Autodesk Fusion 360 part; units mm, degrees
note: some values were not read from the file. Chosen so that the rebuilt part matches the saved one: which bodies a step acts on. Set by a fixed rule: which sketch regions a step uses.
(part 5 of 6)
  point P38 (-7.0016, 32.4227)
  point P39 (-7.9355, 32.3003)
  point P40 (-6.6625, 36.7231)
  point P41 (-7.4801, 35.8372)
  point P42 (-8.2403, 35.0791)
  point P43 (-8.9343, 34.4424)
  point P44 (-7.8535, 39.011)
  point P45 (-9.0481, 38.8495)
  point P46 (-10.1052, 38.6615)
  point P47 (-11.0249, 38.4582)
  point P48 (-10.1422, 42.9752)
  point P49 (-10.8794, 42.0214)
  point P50 (-11.5708, 41.1999)
  point P51 (-12.2066, 40.5051)
  point P52 (-11.5281, 45.1505)
  point P53 (-12.7041, 44.8855)
  point P54 (-13.7407, 44.6061)
  point P55 (-14.6392, 44.3235)
  point P56 (-14.1536, 48.9001)
  point P57 (-14.8049, 47.8857)
  point P58 (-15.422, 47.0071)
  point P59 (-15.9948, 46.2596)
  point P60 (-15.7238, 50.9464)
  point P61 (-16.8722, 50.5799)
  point P62 (-17.8806, 50.2113)
  point P63 (-18.7509, 49.8514)
  point P64 (-18.6661, 54.453)
  point P65 (-19.2265, 53.3857)
  point P66 (-19.7646, 52.4566)
  point P67 (-20.2702, 51.6619)
  point P68 (-20.4086, 56.3546)
  point P69 (-21.5207, 55.8894)
  point P70 (-22.4931, 55.4343)
  point P71 (-23.3289, 54.9999)
  point P72 (-23.6454, 59.5914)
  point P73 (-24.1106, 58.4793)
  point P74 (-24.5657, 57.5069)
  point P75 (-25.0001, 56.6711)
  point P76 (-25.547, 61.3339)
  point P77 (-26.6143, 60.7735)
  point P78 (-27.5434, 60.2354)
  point P79 (-28.3381, 59.7298)
  point P80 (-29.0536, 64.2762)
  point P81 (-29.4201, 63.1278)
  point P82 (-29.7887, 62.1194)
  point P83 (-30.1486, 61.2491)
  point P84 (-31.0999, 65.8464)
  point P85 (-32.1143, 65.1951)
  point P86 (-32.9929, 64.578)
  point P87 (-33.7404, 64.0052)
  point P88 (-34.8495, 68.4719)
  point P89 (-35.1145, 67.2959)
  point P90 (-35.3939, 66.2593)
  point P91 (-35.6765, 65.3608)
  point P92 (-37.0248, 69.8578)
  point P93 (-37.9786, 69.1206)
  point P94 (-38.8001, 68.4292)
  point P95 (-39.4949, 67.7934)
  point P96 (-40.989, 72.1465)
  point P97 (-41.1505, 70.9519)
  point P98 (-41.3385, 69.8948)
  point P99 (-41.5418, 68.9751)
  point P100 (-43.2769, 73.3375)
  point P101 (-44.1628, 72.5199)
  point P102 (-44.9209, 71.7597)
  point P103 (-45.5576, 71.0657)
  point P104 (-47.4254, 75.272)
  point P105 (-47.4822, 74.0678)
  point P106 (-47.5773, 72.9984)
  point P107 (-47.6997, 72.0645)
  point P108 (-49.8084, 76.259)
  point P109 (-50.6197, 75.3674)
  point P110 (-51.3086, 74.5439)
  point P111 (-51.8825, 73.7971)
  point P112 (-54.1098, 77.8246)
  point P113 (-54.0614, 76.6201)
  point P114 (-54.063, 75.5464)
  point P115 (-54.1034, 74.6055)
  point P116 (-56.5697, 78.6002)
  point P117 (-57.3002, 77.6413)
  point P118 (-57.9147, 76.7609)
  point P119 (-58.4213, 75.9669)
  point P120 (-60.9911, 79.7849)
  point P121 (-60.838, 78.5892)
  point P122 (-60.746, 77.5195)
  point P123 (-60.7043, 76.5786)
  point P124 (-63.5093, 80.3432)
  point P125 (-64.1534, 79.3242)
  point P126 (-64.6889, 78.3937)
  point P127 (-65.1244, 77.5585)
  point P128 (-68.0172, 81.1381)
  point P129 (-67.7604, 79.9603)
  point P130 (-67.5755, 78.9026)
  point P131 (-67.452, 77.9689)
  point P132 (-70.5744, 81.4747)
  point P133 (-71.1273, 80.4035)
  point P134 (-71.5796, 79.4298)
  point P135 (-71.9406, 78.5599)
  point P136 (-75.1344, 81.8737)
  point P137 (-74.776, 80.7227)
  point P138 (-74.4996, 79.6853)
  point P139 (-74.2952, 78.7659)
  point P140 (-77.7113, 81.9862)
  point P141 (-78.1687, 80.8709)
  point P142 (-78.5345, 79.8614)
  point P143 (-78.8182, 78.9633)
  point P144 (-82.2887, 81.9862)
  point P145 (-81.8313, 80.8709)
  point P146 (-81.4655, 79.8614)
  point P147 (-81.1818, 78.9633)
  point P148 (-84.8656, 81.8737)
  point P149 (-85.224, 80.7227)
  point P150 (-85.5004, 79.6853)
  point P151 (-85.7048, 78.7659)
  point P152 (-89.4256, 81.4747)
  point P153 (-88.8727, 80.4035)
  point P154 (-88.4204, 79.4298)
  point P155 (-88.0594, 78.5599)
  point P156 (-91.9828, 81.1381)
  point P157 (-92.2396, 79.9603)
  point P158 (-92.4245, 78.9026)
  point P159 (-92.548, 77.9689)
  point P160 (-96.4907, 80.3432)
  point P161 (-95.8466, 79.3242)
  point P162 (-95.3111, 78.3937)
  point P163 (-94.8756, 77.5585)
  point P164 (-99.0089, 79.7849)
  point P165 (-99.162, 78.5892)
  point P166 (-99.254, 77.5195)
  point P167 (-99.2957, 76.5786)
  point P168 (-103.4303, 78.6002)
  point P169 (-102.6998, 77.6413)
  point P170 (-102.0853, 76.7609)
  point P171 (-101.5787, 75.9669)
  point P172 (-105.8902, 77.8246)
  point P173 (-105.9386, 76.6201)
  point P174 (-105.937, 75.5464)
  point P175 (-105.8966, 74.6055)
  point P176 (-110.1916, 76.259)
  point P177 (-109.3803, 75.3674)
  point P178 (-108.6914, 74.5439)
  point P179 (-108.1175, 73.7971)
  point P180 (-112.5746, 75.272)
  point P181 (-112.5178, 74.0678)
  point P182 (-112.4227, 72.9984)
  point P183 (-112.3003, 72.0645)
  point P184 (-116.7231, 73.3375)
  point P185 (-115.8372, 72.5199)
  point P186 (-115.0791, 71.7597)
  point P187 (-114.4424, 71.0657)
  point P188 (-119.011, 72.1465)
  point P189 (-118.8495, 70.9519)
  point P190 (-118.6615, 69.8948)
  point P191 (-118.4582, 68.9751)
  point P192 (-122.9752, 69.8578)
  point P193 (-122.0214, 69.1206)
  point P194 (-121.1999, 68.4292)
  point P195 (-120.5051, 67.7934)
  point P196 (-125.1505, 68.4719)
  point P197 (-124.8855, 67.2959)
  point P198 (-124.6061, 66.2593)
  point P199 (-124.3235, 65.3608)
  point P200 (-128.9001, 65.8464)
  point P201 (-127.8857, 65.1951)
  point P202 (-127.0071, 64.578)
  point P203 (-126.2596, 64.0052)
  point P204 (-130.9464, 64.2762)
  point P205 (-130.5799, 63.1278)
  point P206 (-130.2113, 62.1194)
  point P207 (-129.8514, 61.2491)
  point P208 (-134.453, 61.3339)
  point P209 (-133.3857, 60.7735)
  point P210 (-132.4566, 60.2354)
  point P211 (-131.6619, 59.7298)
  point P212 (-136.3546, 59.5914)
  point P213 (-135.8894, 58.4793)
  point P214 (-135.4343, 57.5069)
  point P215 (-134.9999, 56.6711)
  point P216 (-139.5914, 56.3546)
  point P217 (-138.4793, 55.8894)
  point P218 (-137.5069, 55.4343)
  point P219 (-136.6711, 54.9999)
  point P220 (-141.3339, 54.453)
  point P221 (-140.7735, 53.3857)
  point P222 (-140.2354, 52.4566)
  point P223 (-139.7298, 51.6619)
  point P224 (-144.2762, 50.9464)
  point P225 (-143.1278, 50.5799)
  point P226 (-142.1194, 50.2113)
  point P227 (-141.2491, 49.8514)
  point P228 (-145.8464, 48.9001)
  point P229 (-145.1951, 47.8857)
  point P230 (-144.578, 47.0071)
  point P231 (-144.0052, 46.2596)
  point P232 (-148.4719, 45.1505)
  point P233 (-147.2959, 44.8855)
  point P234 (-146.2593, 44.6061)
  point P235 (-145.3608, 44.3235)
  point P236 (-149.8578, 42.9752)
  point P237 (-149.1206, 42.0214)
  point P238 (-148.4292, 41.1999)
  point P239 (-147.7934, 40.5051)
  point P240 (-152.1465, 39.011)
  point P241 (-150.9519, 38.8495)
  point P242 (-149.8948, 38.6615)
  point P243 (-148.9751, 38.4582)
  point P244 (-153.3375, 36.7231)
  point P245 (-152.5199, 35.8372)
  point P246 (-151.7597, 35.0791)
  point P247 (-151.0657, 34.4424)
  point P248 (-155.272, 32.5746)
  point P249 (-154.0678, 32.5178)
  point P250 (-152.9984, 32.4227)
  point P251 (-152.0645, 32.3003)
  point P252 (-156.259, 30.1916)
  point P253 (-155.3674, 29.3803)
  point P254 (-154.5439, 28.6914)
  point P255 (-153.7971, 28.1175)
  point P256 (-157.8246, 25.8902)
  point P257 (-156.6201, 25.9386)
  point P258 (-155.5464, 25.937)
  point P259 (-154.6055, 25.8966)
  point P260 (-158.6002, 23.4303)
  point P261 (-157.6413, 22.6998)
  point P262 (-156.7609, 22.0853)
  point P263 (-155.9669, 21.5787)
  point P264 (-159.7849, 19.0089)
  point P265 (-158.5892, 19.162)
  point P266 (-157.5195, 19.254)
  point P267 (-156.5786, 19.2957)
  point P268 (-160.3432, 16.4907)
  point P269 (-159.3242, 15.8466)
  point P270 (-158.3937, 15.3111)
  point P271 (-157.5585, 14.8756)
  point P272 (-161.1381, 11.9828)
  point P273 (-159.9603, 12.2396)
  point P274 (-158.9026, 12.4245)
  point P275 (-157.9689, 12.548)
  point P276 (-161.4747, 9.4256)
  point P277 (-160.4035, 8.8727)
  point P278 (-159.4298, 8.4204)
  point P279 (-158.5599, 8.0594)
  point P280 (-161.8737, 4.8656)
  point P281 (-160.7227, 5.224)
  point P282 (-159.6853, 5.5004)
  point P283 (-158.7659, 5.7048)
  point P284 (-161.9862, 2.2887)
  point P285 (-160.8709, 1.8313)
  point P286 (-159.8614, 1.4655)
  point P287 (-158.9633, 1.1818)
  point P288 (-161.9862, -2.2887)
  point P289 (-160.8709, -1.8313)
  point P290 (-159.8614, -1.4655)
  point P291 (-158.9633, -1.1818)
  point P292 (-161.8737, -4.8656)
  point P293 (-160.7227, -5.224)
  point P294 (-159.6853, -5.5004)
  point P295 (-158.7659, -5.7048)
  point P296 (-161.4747, -9.4256)
  point P297 (-160.4035, -8.8727)
  point P298 (-159.4298, -8.4204)
  point P299 (-158.5599, -8.0594)
  point P300 (-161.1381, -11.9828)
  point P301 (-159.9603, -12.2396)
  point P302 (-158.9026, -12.4245)
  point P303 (-157.9689, -12.548)
  point P304 (-160.3432, -16.4907)
  point P305 (-159.3242, -15.8466)
  point P306 (-158.3937, -15.3111)
  point P307 (-157.5585, -14.8756)
  point P308 (-159.7849, -19.0089)
  point P309 (-158.5892, -19.162)
  point P310 (-157.5195, -19.254)
  point P311 (-156.5786, -19.2957)
  point P312 (-158.6002, -23.4303)
  point P313 (-157.6413, -22.6998)
  point P314 (-156.7609, -22.0853)
  point P315 (-155.9669, -21.5787)
  point P316 (-157.8246, -25.8902)
  point P317 (-156.6201, -25.9386)
  point P318 (-155.5464, -25.937)
  point P319 (-154.6055, -25.8966)
  point P320 (-156.259, -30.1916)
  point P321 (-155.3674, -29.3803)
  point P322 (-154.5439, -28.6914)
  point P323 (-153.7971, -28.1175)
  point P324 (-155.272, -32.5746)
  point P325 (-154.0678, -32.5178)
  point P326 (-152.9984, -32.4227)
  point P327 (-152.0645, -32.3003)
  point P328 (-153.3375, -36.7231)
  point P329 (-152.5199, -35.8372)
  point P330 (-151.7597, -35.0791)
  point P331 (-151.0657, -34.4424)
  point P332 (-152.1465, -39.011)
  point P333 (-150.9519, -38.8495)
  point P334 (-149.8948, -38.6615)
  point P335 (-148.9751, -38.4582)
  point P336 (-149.8578, -42.9752)
  point P337 (-149.1206, -42.0214)
  point P338 (-148.4292, -41.1999)
  point P339 (-147.7934, -40.5051)
  point P340 (-148.4719, -45.1505)
  point P341 (-147.2959, -44.8855)
  point P342 (-146.2593, -44.6061)
  point P343 (-145.3608, -44.3235)
  point P344 (-145.8464, -48.9001)
  point P345 (-145.1951, -47.8857)
  point P346 (-144.578, -47.0071)
  point P347 (-144.0052, -46.2596)
  point P348 (-144.2762, -50.9464)
  point P349 (-143.1278, -50.5799)
  point P350 (-142.1194, -50.2113)
  point P351 (-141.2491, -49.8514)
  point P352 (-141.3339, -54.453)
  point P353 (-140.7735, -53.3857)
  point P354 (-140.2354, -52.4566)
  point P355 (-139.7298, -51.6619)
  point P356 (-139.5914, -56.3546)
  point P357 (-138.4793, -55.8894)
  point P358 (-137.5069, -55.4343)
  point P359 (-136.6711, -54.9999)
  point P360 (-136.3546, -59.5914)
  point P361 (-135.8894, -58.4793)
  point P362 (-135.4343, -57.5069)
  point P363 (-134.9999, -56.6711)
  point P364 (-134.453, -61.3339)
  point P365 (-133.3857, -60.7735)
  point P366 (-132.4566, -60.2354)
  point P367 (-131.6619, -59.7298)
  point P368 (-130.9464, -64.2762)
  point P369 (-130.5799, -63.1278)
  point P370 (-130.2113, -62.1194)
  point P371 (-129.8514, -61.2491)
  point P372 (-128.9001, -65.8464)
  point P373 (-127.8857, -65.1951)
  point P374 (-127.0071, -64.578)
  point P375 (-126.2596, -64.0052)
  point P376 (-125.1505, -68.4719)
  point P377 (-124.8855, -67.2959)
  point P378 (-124.6061, -66.2593)
  point P379 (-124.3235, -65.3608)
  point P380 (-122.9752, -69.8578)
  point P381 (-122.0214, -69.1206)
  point P382 (-121.1999, -68.4292)
  point P383 (-120.5051, -67.7934)
  point P384 (-119.011, -72.1465)
  point P385 (-118.8495, -70.9519)
  point P386 (-118.6615, -69.8948)
  point P387 (-118.4582, -68.9751)
  point P388 (-116.7231, -73.3375)
  point P389 (-115.8372, -72.5199)
  point P390 (-115.0791, -71.7597)
  point P391 (-114.4424, -71.0657)
  point P392 (-112.5746, -75.272)
  point P393 (-112.5178, -74.0678)
  point P394 (-112.4227, -72.9984)
  point P395 (-112.3003, -72.0645)
  point P396 (-110.1916, -76.259)
  point P397 (-109.3803, -75.3674)
  point P398 (-108.6914, -74.5439)
  point P399 (-108.1175, -73.7971)
  point P400 (-105.8902, -77.8246)
  point P401 (-105.9386, -76.6201)
  point P402 (-105.937, -75.5464)
  point P403 (-105.8966, -74.6055)
  point P404 (-103.4303, -78.6002)
  point P405 (-102.6998, -77.6413)
  point P406 (-102.0853, -76.7609)
  point P407 (-101.5787, -75.9669)
  point P408 (-99.0089, -79.7849)
  point P409 (-99.162, -78.5892)
  point P410 (-99.254, -77.5195)
  point P411 (-99.2957, -76.5786)
  point P412 (-96.4907, -80.3432)
  point P413 (-95.8466, -79.3242)
  point P414 (-95.3111, -78.3937)
  point P415 (-94.8756, -77.5585)
  point P416 (-91.9828, -81.1381)
  point P417 (-92.2396, -79.9603)
  point P418 (-92.4245, -78.9026)
  point P419 (-92.548, -77.9689)
  point P420 (-89.4256, -81.4747)
  point P421 (-88.8727, -80.4035)
  point P422 (-88.4204, -79.4298)
  point P423 (-88.0594, -78.5599)
  point P424 (-84.8656, -81.8737)
  point P425 (-85.224, -80.7227)
  point P426 (-85.5004, -79.6853)
  point P427 (-85.7048, -78.7659)
  point P428 (-82.2887, -81.9862)
  point P429 (-81.8313, -80.8709)
  point P430 (-81.4655, -79.8614)
  point P431 (-81.1818, -78.9633)
  point P432 (-77.7113, -81.9862)
  point P433 (-78.1687, -80.8709)
  point P434 (-78.5345, -79.8614)
  point P435 (-78.8182, -78.9633)
  point P436 (-75.1344, -81.8737)
  point P437 (-74.776, -80.7227)
  point P438 (-74.4996, -79.6853)
  point P439 (-74.2952, -78.7659)
  point P440 (-70.5744, -81.4747)
  point P441 (-71.1273, -80.4035)
  point P442 (-71.5796, -79.4298)
  point P443 (-71.9406, -78.5599)
  point P444 (-68.0172, -81.1381)
  point P445 (-67.7604, -79.9603)
  point P446 (-67.5755, -78.9026)
  point P447 (-67.452, -77.9689)
  point P448 (-63.5093, -80.3432)
  point P449 (-64.1534, -79.3242)
  point P450 (-64.6889, -78.3937)
  point P451 (-65.1244, -77.5585)
  point P452 (-60.9911, -79.7849)
  point P453 (-60.838, -78.5892)
  point P454 (-60.746, -77.5195)
  point P455 (-60.7043, -76.5786)
  point P456 (-56.5697, -78.6002)
  point P457 (-57.3002, -77.6413)
  point P458 (-57.9147, -76.7609)
  point P459 (-58.4213, -75.9669)
  point P460 (-54.1098, -77.8246)
  point P461 (-54.0614, -76.6201)
  point P462 (-54.063, -75.5464)
  point P463 (-54.1034, -74.6055)
  point P464 (-49.8084, -76.259)
  point P465 (-50.6197, -75.3674)
  point P466 (-51.3086, -74.5439)
  point P467 (-51.8825, -73.7971)
  point P468 (-47.4254, -75.272)
  point P469 (-47.4822, -74.0678)
  point P470 (-47.5773, -72.9984)
  point P471 (-47.6997, -72.0645)
  point P472 (-43.2769, -73.3375)
  point P473 (-44.1628, -72.5199)
  point P474 (-44.9209, -71.7597)
  point P475 (-45.5576, -71.0657)
  point P476 (-40.989, -72.1465)
  point P477 (-41.1505, -70.9519)
  point P478 (-41.3385, -69.8948)
  point P479 (-41.5418, -68.9751)
  point P480 (-37.0248, -69.8578)
  point P481 (-37.9786, -69.1206)
  point P482 (-38.8001, -68.4292)
  point P483 (-39.4949, -67.7934)
  point P484 (-34.8495, -68.4719)
  point P485 (-35.1145, -67.2959)
  point P486 (-35.3939, -66.2593)
  point P487 (-35.6765, -65.3608)
  point P488 (-31.0999, -65.8464)
  point P489 (-32.1143, -65.1951)
  point P490 (-32.9929, -64.578)
  point P491 (-33.7404, -64.0052)
  point P492 (-29.0536, -64.2762)
  point P493 (-29.4201, -63.1278)
  point P494 (-29.7887, -62.1194)
  point P495 (-30.1486, -61.2491)
  point P496 (-25.547, -61.3339)
  point P497 (-26.6143, -60.7735)
  point P498 (-27.5434, -60.2354)
  point P499 (-28.3381, -59.7298)
  point P500 (-23.6454, -59.5914)
  point P501 (-24.1106, -58.4793)
  point P502 (-24.5657, -57.5069)
  point P503 (-25.0001, -56.6711)
  point P504 (-20.4086, -56.3546)
  point P505 (-21.5207, -55.8894)
  point P506 (-22.4931, -55.4343)
  point P507 (-23.3289, -54.9999)
  point P508 (-18.6661, -54.453)
  point P509 (-19.2265, -53.3857)
  point P510 (-19.7646, -52.4566)
  point P511 (-20.2702, -51.6619)
  point P512 (-15.7238, -50.9464)
  point P513 (-16.8722, -50.5799)
  point P514 (-17.8806, -50.2113)
  point P515 (-18.7509, -49.8514)
  point P516 (-14.1536, -48.9001)
  point P517 (-14.8049, -47.8857)
  point P518 (-15.422, -47.0071)
  point P519 (-15.9948, -46.2596)
  point P520 (-11.5281, -45.1505)
  point P521 (-12.7041, -44.8855)
  point P522 (-13.7407, -44.6061)
  point P523 (-14.6392, -44.3235)
  point P524 (-10.1422, -42.9752)
  point P525 (-10.8794, -42.0214)
  point P526 (-11.5708, -41.1999)
  point P527 (-12.2066, -40.5051)
  point P528 (-7.8535, -39.011)
  point P529 (-9.0481, -38.8495)
  point P530 (-10.1052, -38.6615)
  point P531 (-11.0249, -38.4582)
  point P532 (-6.6625, -36.7231)
  point P533 (-7.4801, -35.8372)
  point P534 (-8.2403, -35.0791)
  point P535 (-8.9343, -34.4424)
  point P536 (-4.728, -32.5746)
  point P537 (-5.9322, -32.5178)
  point P538 (-7.0016, -32.4227)
  point P539 (-7.9355, -32.3003)
  point P540 (-3.741, -30.1916)
  point P541 (-4.6326, -29.3803)
  point P542 (-5.4561, -28.6914)
  point P543 (-6.2029, -28.1175)
  point P544 (-2.1754, -25.8902)
  point P545 (-3.3799, -25.9386)
  point P546 (-4.4536, -25.937)
  point P547 (-5.3945, -25.8966)
  point P548 (-1.3998, -23.4303)
  point P549 (-2.3587, -22.6998)
  point P550 (-3.2391, -22.0853)
  point P551 (-4.0331, -21.5787)
  point P552 (-0.2151, -19.0089)
  point P553 (-1.4108, -19.162)
  point P554 (-2.4805, -19.254)
  point P555 (-3.4214, -19.2957)
  point P556 (0.3432, -16.4907)
  point P557 (-0.6758, -15.8466)
  point P558 (-1.6063, -15.3111)
  point P559 (-2.4415, -14.8756)
  point P560 (1.1381, -11.9828)
  point P561 (-0.0397, -12.2396)
  point P562 (-1.0974, -12.4245)
  point P563 (-2.0311, -12.548)
  point P564 (1.4747, -9.4256)
  point P565 (0.4035, -8.8727)
  point P566 (-0.5702, -8.4204)
  point P567 (-1.4401, -8.0594)
  point P568 (1.8737, -4.8656)
  point P569 (0.7227, -5.224)
  point P570 (-0.3147, -5.5004)
  point P571 (-1.2341, -5.7048)
  point P572 (1.9862, -2.2887)
  point P573 (0.8709, -1.8313)
  point P574 (-0.1386, -1.4655)
  point P575 (-1.0367, -1.1818)
extrude "押し出し1'''''''''''''''" add sketch "スケッチ1 (16)" along normal blind 16 from surface at 66 separate body contours S0 A0 S1 A1 S2 A2 S3 A3 S4 A4 S5 A5 S6 A6 S7 A7 S8 A8 S9 A9 S10 A10 S11 A11 S12 A12 S13 A13 S14 A14 S15 A15 S16 A16 S17 A17 S18 A18 S19 A19 S20 A20 S21 A21 S22 A22 S23 A23 S24 A24 S25 A25 S26 A26 S27 A27 S28 A28 S29 A29 S30 A30 S31 A31 S32 A32 S33 A33 S34 A34 S35 A35 S36 A36 S37 A37 S38 A38 S39 A39 S40 A40 S41 A41 S42 A42 S43 A43 S44 A44 S45 A45 S46 A46 S47 A47 S48 A48 S49 A49 S50 A50 S51 A51 S52 A52 S53 A53 S54 A54 S55 A55 S56 A56 S57 A57 S58 A58 S59 A59 S60 A60 S61 A61 S62 A62 S63 A63 S64 A64 S65 A65 S66 A66 S67 A67 S68 A68 S69 A69 S70 A70 S71 A71 S72 A72 S73 A73 S74 A74 S75 A75 S76 A76 S77 A77 S78 A78 S79 A79 S80 A80 S81 A81 S82 A82 S83 A83 S84 A84 S85 A85 S86 A86 S87 A87 S88 A88 S89 A89 S90 A90 S91 A91 S92 A92 S93 A93 S94 A94 S95 A95 S96 A96 S97 A97 S98 A98 S99 A99 S100 A100 S101 A101 S102 A102 S103 A103 S104 A104 S105 A105 S106 A106 S107 A107 S108 A108 S109 A109 S110 A110 S111 A111 S112 A112 S113 A113 S114 A114 S115 A115 S116 A116 S117 A117 S118 A118 S119 A119 S120 A120 S121 A121 S122 A122 S123 A123 S124 A124 S125 A125 S126 A126 S127 A127 S128 A128 S129 A129 S130 A130 S131 A131 S132 A132 S133 A133 S134 A134 S135 A135 S136 A136 S137 A137 S138 A138 S139 A139 S140 A140 S141 A141 S142 A142 S143 A143 makes body 24 in component "Intermediate_Spur_Gear_72T"
sketch "スケッチ2 (15)" plane through (0, 0, 0) normal (0, 0, 1) x (1, 0, 0) in component "Intermediate_Spur_Gear_72T"
  circle A0 centre (-80, 0) radius 70
  circle A1 centre (-80, 0) radius 30
extrude "押し出し2''''''''''''''" cut sketch "スケッチ2 (15)" along normal blind 5 from surface at 78 bodies 24 in component "Intermediate_Spur_Gear_72T"
sketch "スケッチ3 (14)" plane through (0, 0, 0) normal (0, 0, 1) x (1, 0, 0) in component "Intermediate_Spur_Gear_72T"
  circle A0 centre (-80, 0) radius 70
  circle A1 centre (-80, 0) radius 30
sketch "スケッチ4 (9)" plane through (0, 0, 0) normal (0, 0, 1) x (1, 0, 0) in component "Intermediate_Spur_Gear_72T"
  circle A0 centre (-36.6987, 25) radius 19
  circle A1 centre (-80, 50) radius 19
  circle A2 centre (-123.3013, 25) radius 19
  circle A3 centre (-123.3013, -25) radius 19
  circle A4 centre (-80, -50) radius 19
  circle A5 centre (-36.6987, -25) radius 19
extrude "押し出し4'''''''" cut sketch "スケッチ4 (9)" along normal blind 24 from surface at 62 bodies 24 in component "Intermediate_Spur_Gear_72T"
sketch "スケッチ5 (7)" plane through (0, 0, 0) normal (0, 0, 1) x (1, 0, 0) in component "Intermediate_Spur_Gear_72T"
  circle A0 centre (-80, 0) radius 8
extrude "押し出し5'''''" cut sketch "スケッチ5 (7)" along normal blind 24 from surface at 62 bodies 24 in component "Intermediate_Spur_Gear_72T"
sketch "スケッチ1 (17)" plane through (0, 0, 0) normal (0, 0, 1) x (1, 0, 0) in component "Intermediate_Pinion_12T"
  spline S0 degree 5 poles (-1.2395, 0.5747) (-1.2073, 0.5961) (-1.143, 0.6386) (-1.0472, 0.7007) (-0.9206, 0.7807) (-0.7642, 0.8756) (-0.6097, 0.9657) (-0.457, 1.0507) (-0.3062, 1.1306) (-0.1569, 1.2054) (-0.0092, 1.2751) (0.1373, 1.3396) (0.2823, 1.3989) (0.4255, 1.453) (0.5663, 1.5022) (0.7033, 1.5465) (0.8353, 1.5862) (0.9609, 1.6214) (1.0797, 1.6523) (1.1919, 1.6789) (1.2996, 1.7011) (1.4047, 1.7185) (1.5082, 1.7313) (1.609, 1.7398) (1.7017, 1.7448) (1.7783, 1.7477) (1.8329, 1.7495) (1.865, 1.7509) (1.8842, 1.7511) (1.9081, 1.7485) (1.9564, 1.7413) (2.0459, 1.7278) (2.1885, 1.7069) (2.3925, 1.6777) (2.6632, 1.6398) (3.0034, 1.5929) (3.3322, 1.5482) (3.6107, 1.5105) (3.8106, 1.4836) (3.914, 1.4697) knots 0 0 0 0 0 0 0.028571 0.057143 0.085714 0.114286 0.142857 0.171429 0.2 0.228571 0.257143 0.285714 0.314286 0.342857 0.371429 0.4 0.428571 0.457143 0.485714 0.514286 0.542857 0.571429 0.6 0.628571 0.657143 0.685714 0.714286 0.742857 0.771429 0.8 0.828571 0.857143 0.885714 0.914286 0.942857 0.971429 1 1 1 1 1 1
  arc A0 (3.914, 1.4697) -> (-1.2395, -0.5747) centre (1.6081, -0.2353) ccw
  spline S1 degree 5 poles (-1.2395, -0.5747) (-1.2073, -0.5961) (-1.143, -0.6386) (-1.0472, -0.7007) (-0.9206, -0.7807) (-0.7642, -0.8756) (-0.6097, -0.9657) (-0.457, -1.0507) (-0.3062, -1.1306) (-0.1569, -1.2054) (-0.0092, -1.2751) (0.1373, -1.3396) (0.2823, -1.3989) (0.4255, -1.453) (0.5663, -1.5022) (0.7033, -1.5465) (0.8353, -1.5862) (0.9609, -1.6214) (1.0797, -1.6523) (1.1919, -1.6789) (1.2996, -1.7011) (1.4047, -1.7185) (1.5082, -1.7313) (1.609, -1.7398) (1.7017, -1.7448) (1.7783, -1.7477) (1.8329, -1.7495) (1.865, -1.7509) (1.8842, -1.7511) (1.9081, -1.7485) (1.9564, -1.7413) (2.0459, -1.7278) (2.1885, -1.7069) (2.3925, -1.6777) (2.6632, -1.6398) (3.0034, -1.5929) (3.3322, -1.5482) (3.6107, -1.5105) (3.8106, -1.4836) (3.914, -1.4697) knots 0 0 0 0 0 0 0.028571 0.057143 0.085714 0.114286 0.142857 0.171429 0.2 0.228571 0.257143 0.285714 0.314286 0.342857 0.371429 0.4 0.428571 0.457143 0.485714 0.514286 0.542857 0.571429 0.6 0.628571 0.657143 0.685714 0.714286 0.742857 0.771429 0.8 0.828571 0.857143 0.885714 0.914286 0.942857 0.971429 1 1 1 1 1 1
  arc A1 (0.5818, -7.3721) -> (3.914, -1.4697) centre (-0.2795, -2.994) ccw
  spline S2 degree 5 poles (0.5818, -7.3721) (0.599, -7.3374) (0.6335, -7.2685) (0.6854, -7.1668) (0.7551, -7.0342) (0.843, -6.8738) (0.9318, -6.7185) (1.0215, -6.5686) (1.1122, -6.4239) (1.204, -6.2845) (1.2972, -6.1503) (1.3917, -6.0213) (1.4876, -5.8974) (1.5846, -5.7789) (1.6819, -5.6659) (1.7785, -5.559) (1.8729, -5.4587) (1.9641, -5.3653) (2.0515, -5.2792) (2.1354, -5.2) (2.2175, -5.127) (2.2998, -5.0594) (2.3831, -4.9965) (2.4662, -4.9388) (2.5439, -4.8881) (2.6088, -4.8473) (2.6552, -4.8184) (2.6823, -4.8012) (2.6989, -4.7914) (2.7208, -4.7817) (2.7663, -4.7638) (2.8505, -4.7307) (2.9845, -4.6776) (3.1758, -4.6008) (3.4291, -4.4983) (3.7472, -4.3688) (4.0543, -4.2431) (4.3143, -4.1365) (4.5009, -4.0599) (4.5974, -4.0202) knots 0 0 0 0 0 0 0.028571 0.057143 0.085714 0.114286 0.142857 0.171429 0.2 0.228571 0.257143 0.285714 0.314286 0.342857 0.371429 0.4 0.428571 0.457143 0.485714 0.514286 0.542857 0.571429 0.6 0.628571 0.657143 0.685714 0.714286 0.742857 0.771429 0.8 0.828571 0.857143 0.885714 0.914286 0.942857 0.971429 1 1 1 1 1 1
  arc A2 (4.5974, -4.0202) -> (1.1565, -8.3674) centre (3.4529, -6.6497) ccw
  spline S3 degree 5 poles (1.1565, -8.3674) (1.1952, -8.3699) (1.272, -8.3745) (1.3861, -8.3804) (1.5357, -8.3863) (1.7187, -8.3904) (1.8975, -8.3911) (2.0722, -8.3884) (2.2428, -8.3822) (2.4094, -8.3724) (2.5723, -8.3588) (2.7313, -8.3415) (2.8865, -8.3203) (3.0377, -8.2956) (3.1841, -8.2678) (3.325, -8.2376) (3.4591, -8.206) (3.5855, -8.1737) (3.7038, -8.1411) (3.8143, -8.108) (3.9186, -8.0734) (4.0184, -8.036) (4.1145, -7.9953) (4.206, -7.9522) (4.2887, -7.9102) (4.3565, -7.8744) (4.4048, -7.8487) (4.4332, -7.8338) (4.45, -7.8243) (4.4694, -7.8102) (4.5076, -7.7798) (4.5783, -7.7234) (4.6914, -7.6339) (4.8535, -7.5067) (5.0689, -7.3385) (5.3401, -7.1278) (5.6025, -6.9247) (5.8248, -6.7528) (5.9845, -6.6295) (6.0671, -6.5658) knots 0 0 0 0 0 0 0.028571 0.057143 0.085714 0.114286 0.142857 0.171429 0.2 0.228571 0.257143 0.285714 0.314286 0.342857 0.371429 0.4 0.428571 0.457143 0.485714 0.514286 0.542857 0.571429 0.6 0.628571 0.657143 0.685714 0.714286 0.742857 0.771429 0.8 0.828571 0.857143 0.885714 0.914286 0.942857 0.971429 1 1 1 1 1 1
  arc A3 (6.1326, -13.3435) -> (6.0671, -6.5658) centre (3.1976, -9.9826) ccw
  spline S4 degree 5 poles (6.1326, -13.3435) (6.1301, -13.3048) (6.1255, -13.228) (6.1196, -13.1139) (6.1137, -12.9643) (6.1096, -12.7813) (6.1089, -12.6025) (6.1116, -12.4278) (6.1178, -12.2572) (6.1276, -12.0906) (6.1412, -11.9277) (6.1585, -11.7687) (6.1797, -11.6135) (6.2044, -11.4623) (6.2322, -11.3159) (6.2624, -11.175) (6.294, -11.0409) (6.3263, -10.9145) (6.3589, -10.7962) (6.392, -10.6857) (6.4266, -10.5814) (6.464, -10.4816) (6.5047, -10.3855) (6.5478, -10.294) (6.5898, -10.2113) (6.6256, -10.1435) (6.6513, -10.0952) (6.6662, -10.0668) (6.6757, -10.05) (6.6898, -10.0306) (6.7202, -9.9924) (6.7766, -9.9217) (6.8661, -9.8086) (6.9933, -9.6465) (7.1615, -9.4311) (7.3722, -9.1599) (7.5753, -8.8975) (7.7472, -8.6752) (7.8705, -8.5155) (7.9342, -8.4329) knots 0 0 0 0 0 0 0.028571 0.057143 0.085714 0.114286 0.142857 0.171429 0.2 0.228571 0.257143 0.285714 0.314286 0.342857 0.371429 0.4 0.428571 0.457143 0.485714 0.514286 0.542857 0.571429 0.6 0.628571 0.657143 0.685714 0.714286 0.742857 0.771429 0.8 0.828571 0.857143 0.885714 0.914286 0.942857 0.971429 1 1 1 1 1 1
  arc A4 (7.9342, -8.4329) -> (7.1279, -13.9182) centre (8.2578, -11.2823) ccw
  spline S5 degree 5 poles (7.1279, -13.9182) (7.1626, -13.901) (7.2315, -13.8665) (7.3332, -13.8146) (7.4658, -13.7449) (7.6262, -13.657) (7.7815, -13.5682) (7.9314, -13.4785) (8.0761, -13.3878) (8.2155, -13.296) (8.3497, -13.2028) (8.4787, -13.1083) (8.6026, -13.0124) (8.7211, -12.9154) (8.8341, -12.8181) (8.941, -12.7215) (9.0413, -12.6271) (9.1347, -12.5359) (9.2208, -12.4485) (9.3, -12.3646) (9.373, -12.2825) (9.4406, -12.2002) (9.5035, -12.1169) (9.5612, -12.0338) (9.6119, -11.9561) (9.6527, -11.8912) (9.6816, -11.8448) (9.6988, -11.8177) (9.7086, -11.8011) (9.7183, -11.7792) (9.7362, -11.7337) (9.7693, -11.6495) (9.8224, -11.5155) (9.8992, -11.3242) (10.0017, -11.0709) (10.1312, -10.7528) (10.2569, -10.4457) (10.3635, -10.1857) (10.4401, -9.9991) (10.4798, -9.9026) knots 0 0 0 0 0 0 0.028571 0.057143 0.085714 0.114286 0.142857 0.171429 0.2 0.228571 0.257143 0.285714 0.314286 0.342857 0.371429 0.4 0.428571 0.457143 0.485714 0.514286 0.542857 0.571429 0.6 0.628571 0.657143 0.685714 0.714286 0.742857 0.771429 0.8 0.828571 0.857143 0.885714 0.914286 0.942857 0.971429 1 1 1 1 1 1
  arc A5 (13.9253, -15.7395) -> (10.4798, -9.9026) centre (9.7032, -14.2964) ccw
  spline S6 degree 5 poles (13.9253, -15.7395) (13.9039, -15.7073) (13.8614, -15.643) (13.7993, -15.5472) (13.7193, -15.4206) (13.6244, -15.2642) (13.5343, -15.1097) (13.4493, -14.957) (13.3694, -14.8062) (13.2946, -14.6569) (13.2249, -14.5092) (13.1604, -14.3627) (13.1011, -14.2177) (13.047, -14.0745) (12.9978, -13.9337) (12.9535, -13.7967) (12.9138, -13.6647) (12.8786, -13.5391) (12.8477, -13.4203) (12.8211, -13.3081) (12.7989, -13.2004) (12.7815, -13.0953) (12.7687, -12.9918) (12.7602, -12.891) (12.7552, -12.7983) (12.7523, -12.7217) (12.7505, -12.6671) (12.7491, -12.635) (12.7489, -12.6158) (12.7515, -12.5919) (12.7587, -12.5436) (12.7722, -12.4541) (12.7931, -12.3115) (12.8223, -12.1075) (12.8602, -11.8368) (12.9071, -11.4966) (12.9518, -11.1678) (12.9895, -10.8893) (13.0164, -10.6894) (13.0303, -10.586) knots 0 0 0 0 0 0 0.028571 0.057143 0.085714 0.114286 0.142857 0.171429 0.2 0.228571 0.257143 0.285714 0.314286 0.342857 0.371429 0.4 0.428571 0.457143 0.485714 0.514286 0.542857 0.571429 0.6 0.628571 0.657143 0.685714 0.714286 0.742857 0.771429 0.8 0.828571 0.857143 0.885714 0.914286 0.942857 0.971429 1 1 1 1 1 1
  arc A6 (13.0303, -10.586) -> (15.0747, -15.7395) centre (14.7353, -12.8919) ccw
  spline S7 degree 5 poles (15.0747, -15.7395) (15.0961, -15.7073) (15.1386, -15.643) (15.2007, -15.5472) (15.2807, -15.4206) (15.3756, -15.2642) (15.4657, -15.1097) (15.5507, -14.957) (15.6306, -14.8062) (15.7054, -14.6569) (15.7751, -14.5092) (15.8396, -14.3627) (15.8989, -14.2177) (15.953, -14.0745) (16.0022, -13.9337) (16.0465, -13.7967) (16.0862, -13.6647) (16.1214, -13.5391) (16.1523, -13.4203) (16.1789, -13.3081) (16.2011, -13.2004) (16.2185, -13.0953) (16.2313, -12.9918) (16.2398, -12.891) (16.2448, -12.7983) (16.2477, -12.7217) (16.2495, -12.6671) (16.2509, -12.635) (16.2511, -12.6158) (16.2485, -12.5919) (16.2413, -12.5436) (16.2278, -12.4541) (16.2069, -12.3115) (16.1777, -12.1075) (16.1398, -11.8368) (16.0929, -11.4966) (16.0482, -11.1678) (16.0105, -10.8893) (15.9836, -10.6894) (15.9697, -10.586) knots 0 0 0 0 0 0 0.028571 0.057143 0.085714 0.114286 0.142857 0.171429 0.2 0.228571 0.257143 0.285714 0.314286 0.342857 0.371429 0.4 0.428571 0.457143 0.485714 0.514286 0.542857 0.571429 0.6 0.628571 0.657143 0.685714 0.714286 0.742857 0.771429 0.8 0.828571 0.857143 0.885714 0.914286 0.942857 0.971429 1 1 1 1 1 1
  arc A7 (21.8721, -13.9182) -> (15.9697, -10.586) centre (17.494, -14.7795) ccw
  spline S8 degree 5 poles (21.8721, -13.9182) (21.8374, -13.901) (21.7685, -13.8665) (21.6668, -13.8146) (21.5342, -13.7449) (21.3738, -13.657) (21.2185, -13.5682) (21.0686, -13.4785) (20.9239, -13.3878) (20.7845, -13.296) (20.6503, -13.2028) (20.5213, -13.1083) (20.3974, -13.0124) (20.2789, -12.9154) (20.1659, -12.8181) (20.059, -12.7215) (19.9587, -12.6271) (19.8653, -12.5359) (19.7792, -12.4485) (19.7, -12.3646) (19.627, -12.2825) (19.5594, -12.2002) (19.4965, -12.1169) (19.4388, -12.0338) (19.3881, -11.9561) (19.3473, -11.8912) (19.3184, -11.8448) (19.3012, -11.8177) (19.2914, -11.8011) (19.2817, -11.7792) (19.2638, -11.7337) (19.2307, -11.6495) (19.1776, -11.5155) (19.1008, -11.3242) (18.9983, -11.0709) (18.8688, -10.7528) (18.7431, -10.4457) (18.6365, -10.1857) (18.5599, -9.9991) (18.5202, -9.9026) knots 0 0 0 0 0 0 0.028571 0.057143 0.085714 0.114286 0.142857 0.171429 0.2 0.228571 0.257143 0.285714 0.314286 0.342857 0.371429 0.4 0.428571 0.457143 0.485714 0.514286 0.542857 0.571429 0.6 0.628571 0.657143 0.685714 0.714286 0.742857 0.771429 0.8 0.828571 0.857143 0.885714 0.914286 0.942857 0.971429 1 1 1 1 1 1
  arc A8 (18.5202, -9.9026) -> (22.8674, -13.3435) centre (21.1497, -11.0471) ccw
  spline S9 degree 5 poles (22.8674, -13.3435) (22.8699, -13.3048) (22.8745, -13.228) (22.8804, -13.1139) (22.8863, -12.9643) (22.8904, -12.7813) (22.8911, -12.6025) (22.8884, -12.4278) (22.8822, -12.2572) (22.8724, -12.0906) (22.8588, -11.9277) (22.8415, -11.7687) (22.8203, -11.6135) (22.7956, -11.4623) (22.7678, -11.3159) (22.7376, -11.175) (22.706, -11.0409) (22.6737, -10.9145) (22.6411, -10.7962) (22.608, -10.6857) (22.5734, -10.5814) (22.536, -10.4816) (22.4953, -10.3855) (22.4522, -10.294) (22.4102, -10.2113) (22.3744, -10.1435) (22.3487, -10.0952) (22.3338, -10.0668) (22.3243, -10.05) (22.3102, -10.0306) (22.2798, -9.9924) (22.2234, -9.9217) (22.1339, -9.8086) (22.0067, -9.6465) (21.8385, -9.4311) (21.6278, -9.1599) (21.4247, -8.8975) (21.2528, -8.6752) (21.1295, -8.5155) (21.0658, -8.4329) knots 0 0 0 0 0 0 0.028571 0.057143 0.085714 0.114286 0.142857 0.171429 0.2 0.228571 0.257143 0.285714 0.314286 0.342857 0.371429 0.4 0.428571 0.457143 0.485714 0.514286 0.542857 0.571429 0.6 0.628571 0.657143 0.685714 0.714286 0.742857 0.771429 0.8 0.828571 0.857143 0.885714 0.914286 0.942857 0.971429 1 1 1 1 1 1
  arc A9 (27.8435, -8.3674) -> (21.0658, -8.4329) centre (24.4826, -11.3024) ccw
  spline S10 degree 5 poles (27.8435, -8.3674) (27.8048, -8.3699) (27.728, -8.3745) (27.6139, -8.3804) (27.4643, -8.3863) (27.2813, -8.3904) (27.1025, -8.3911) (26.9278, -8.3884) (26.7572, -8.3822) (26.5906, -8.3724) (26.4277, -8.3588) (26.2687, -8.3415) (26.1135, -8.3203) (25.9623, -8.2956) (25.8159, -8.2678) (25.675, -8.2376) (25.5409, -8.206) (25.4145, -8.1737) (25.2962, -8.1411) (25.1857, -8.108) (25.0814, -8.0734) (24.9816, -8.036) (24.8855, -7.9953) (24.794, -7.9522) (24.7113, -7.9102) (24.6435, -7.8744) (24.5952, -7.8487) (24.5668, -7.8338) (24.55, -7.8243) (24.5306, -7.8102) (24.4924, -7.7798) (24.4217, -7.7234) (24.3086, -7.6339) (24.1465, -7.5067) (23.9311, -7.3385) (23.6599, -7.1278) (23.3975, -6.9247) (23.1752, -6.7528) (23.0155, -6.6295) (22.9329, -6.5658) knots 0 0 0 0 0 0 0.028571 0.057143 0.085714 0.114286 0.142857 0.171429 0.2 0.228571 0.257143 0.285714 0.314286 0.342857 0.371429 0.4 0.428571 0.457143 0.485714 0.514286 0.542857 0.571429 0.6 0.628571 0.657143 0.685714 0.714286 0.742857 0.771429 0.8 0.828571 0.857143 0.885714 0.914286 0.942857 0.971429 1 1 1 1 1 1
  arc A10 (22.9329, -6.5658) -> (28.4182, -7.3721) centre (25.7823, -6.2422) ccw
  spline S11 degree 5 poles (28.4182, -7.3721) (28.401, -7.3374) (28.3665, -7.2685) (28.3146, -7.1668) (28.2449, -7.0342) (28.157, -6.8738) (28.0682, -6.7185) (27.9785, -6.5686) (27.8878, -6.4239) (27.796, -6.2845) (27.7028, -6.1503) (27.6083, -6.0213) (27.5124, -5.8974) (27.4154, -5.7789) (27.3181, -5.6659) (27.2215, -5.559) (27.1271, -5.4587) (27.0359, -5.3653) (26.9485, -5.2792) (26.8646, -5.2) (26.7825, -5.127) (26.7002, -5.0594) (26.6169, -4.9965) (26.5338, -4.9388) (26.4561, -4.8881) (26.3912, -4.8473) (26.3448, -4.8184) (26.3177, -4.8012) (26.3011, -4.7914) (26.2792, -4.7817) (26.2337, -4.7638) (26.1495, -4.7307) (26.0155, -4.6776) (25.8242, -4.6008) (25.5709, -4.4983) (25.2528, -4.3688) (24.9457, -4.2431) (24.6857, -4.1365) (24.4991, -4.0599) (24.4026, -4.0202) knots 0 0 0 0 0 0 0.028571 0.057143 0.085714 0.114286 0.142857 0.171429 0.2 0.228571 0.257143 0.285714 0.314286 0.342857 0.371429 0.4 0.428571 0.457143 0.485714 0.514286 0.542857 0.571429 0.6 0.628571 0.657143 0.685714 0.714286 0.742857 0.771429 0.8 0.828571 0.857143 0.885714 0.914286 0.942857 0.971429 1 1 1 1 1 1
  arc A11 (30.2395, -0.5747) -> (24.4026, -4.0202) centre (28.7964, -4.7968) ccw
  spline S12 degree 5 poles (30.2395, -0.5747) (30.2073, -0.5961) (30.143, -0.6386) (30.0472, -0.7007) (29.9206, -0.7807) (29.7642, -0.8756) (29.6097, -0.9657) (29.457, -1.0507) (29.3062, -1.1306) (29.1569, -1.2054) (29.0092, -1.2751) (28.8627, -1.3396) (28.7177, -1.3989) (28.5745, -1.453) (28.4337, -1.5022) (28.2967, -1.5465) (28.1647, -1.5862) (28.0391, -1.6214) (27.9203, -1.6523) (27.8081, -1.6789) (27.7004, -1.7011) (27.5953, -1.7185) (27.4918, -1.7313) (27.391, -1.7398) (27.2983, -1.7448) (27.2217, -1.7477) (27.1671, -1.7495) (27.135, -1.7509) (27.1158, -1.7511) (27.0919, -1.7485) (27.0436, -1.7413) (26.9541, -1.7278) (26.8115, -1.7069) (26.6075, -1.6777) (26.3368, -1.6398) (25.9966, -1.5929) (25.6678, -1.5482) (25.3893, -1.5105) (25.1894, -1.4836) (25.086, -1.4697) knots 0 0 0 0 0 0 0.028571 0.057143 0.085714 0.114286 0.142857 0.171429 0.2 0.228571 0.257143 0.285714 0.314286 0.342857 0.371429 0.4 0.428571 0.457143 0.485714 0.514286 0.542857 0.571429 0.6 0.628571 0.657143 0.685714 0.714286 0.742857 0.771429 0.8 0.828571 0.857143 0.885714 0.914286 0.942857 0.971429 1 1 1 1 1 1
  arc A12 (25.086, -1.4697) -> (30.2395, 0.5747) centre (27.3919, 0.2353) ccw
  spline S13 degree 5 poles (30.2395, 0.5747) (30.2073, 0.5961) (30.143, 0.6386) (30.0472, 0.7007) (29.9206, 0.7807) (29.7642, 0.8756) (29.6097, 0.9657) (29.457, 1.0507) (29.3062, 1.1306) (29.1569, 1.2054) (29.0092, 1.2751) (28.8627, 1.3396) (28.7177, 1.3989) (28.5745, 1.453) (28.4337, 1.5022) (28.2967, 1.5465) (28.1647, 1.5862) (28.0391, 1.6214) (27.9203, 1.6523) (27.8081, 1.6789) (27.7004, 1.7011) (27.5953, 1.7185) (27.4918, 1.7313) (27.391, 1.7398) (27.2983, 1.7448) (27.2217, 1.7477) (27.1671, 1.7495) (27.135, 1.7509) (27.1158, 1.7511) (27.0919, 1.7485) (27.0436, 1.7413) (26.9541, 1.7278) (26.8115, 1.7069) (26.6075, 1.6777) (26.3368, 1.6398) (25.9966, 1.5929) (25.6678, 1.5482) (25.3893, 1.5105) (25.1894, 1.4836) (25.086, 1.4697) knots 0 0 0 0 0 0 0.028571 0.057143 0.085714 0.114286 0.142857 0.171429 0.2 0.228571 0.257143 0.285714 0.314286 0.342857 0.371429 0.4 0.428571 0.457143 0.485714 0.514286 0.542857 0.571429 0.6 0.628571 0.657143 0.685714 0.714286 0.742857 0.771429 0.8 0.828571 0.857143 0.885714 0.914286 0.942857 0.971429 1 1 1 1 1 1
  arc A13 (28.4182, 7.3721) -> (25.086, 1.4697) centre (29.2795, 2.994) ccw